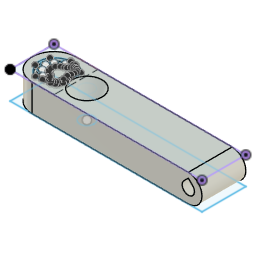
paw v9 (Autodesk Fusion 360 design; units mm, degrees)
Autodesk Fusion 360 part; units mm, degrees
note: some values were not read from the file. Set by a fixed rule: which sketch regions a step uses.
sketch "Sketch1" plane through (0, 0, 0) normal (0, 0, 1) x (1, 0, 0)
  line L0 (-0.0918, 15) -> (34.9082, 15)
  line L1 (34.9082, 15) -> (34.9082, 7)
  line L2 (34.9082, 7) -> (-0.0918, 7)
  line L3 (-0.0918, 7) -> (-0.0918, 15)
  circle A0 centre (9.9082, 11) radius 1.25
  dimension "d1" = 35
  dimension "d2" = 8
  dimension "d3" = 2.5
  dimension "d4" = 25
  dimension "d5" = 4
  constraint horizontal L0
  constraint vertical L1
  constraint horizontal L2
  constraint vertical L3
  measures "d1" distance of L0.start L0.end
  measures "d2" distance of L0.start L2.end
  measures "d3" diameter of A0
  measures "d4" distance of L1 A0.centre
  measures "d5" distance of L0 A0.centre
extrude "Extrude1" add sketch "Sketch1" along normal blind 5
sketch "Sketch2" plane through (0, 0, 5) normal (0, 0, 1) x (-1, 0, 0)
  circle A0 centre (-9.9082, -11) radius 1.25
  spline S0 degree 5 poles (-6.6668, -9.044) (-6.6524, -9.0222) (-6.6233, -8.9806) (-6.5785, -8.9237) (-6.5167, -8.8567) (-6.4345, -8.7811) (-6.3432, -8.7078) (-6.2367, -8.6364) (-6.1068, -8.5717) (-5.9478, -8.5207) (-5.758, -8.4891) (-5.5438, -8.4783) (-5.3207, -8.4835) (-5.1077, -8.496) (-4.922, -8.5058) (-4.7747, -8.5033) (-4.6652, -8.4819) (-4.5768, -8.44) (-4.4867, -8.38) (-4.3721, -8.3084) (-4.22, -8.2356) (-4.0277, -8.1741) (-3.7993, -8.1372) (-3.5437, -8.1373) (-3.272, -8.1841) (-2.9948, -8.2832) (-2.7204, -8.4347) (-2.4559, -8.635) (-2.207, -8.8773) (-1.9783, -9.1532) (-1.7741, -9.4534) (-1.5979, -9.7688) (-1.4537, -10.0915) (-1.3454, -10.416) (-1.2774, -10.7396) (-1.2539, -11.0611) (-1.2785, -11.3805) (-1.3538, -11.6979) (-1.4808, -12.0127) (-1.6588, -12.323) (-1.8844, -12.6248) (-2.1518, -12.911) (-2.4522, -13.1718) (-2.775, -13.3969) (-3.1086, -13.5764) (-3.4406, -13.7026) (-3.7589, -13.7713) (-4.0521, -13.7834) (-4.3104, -13.7462) (-4.5259, -13.6756) (-4.694, -13.5945) (-4.8153, -13.5267) (-4.8979, -13.4912) (-4.9591, -13.4967) (-5.0282, -13.5353) (-5.1366, -13.588) (-5.3079, -13.6318) (-5.5459, -13.6462) (-5.8352, -13.6163) (-6.1489, -13.5318) (-6.4539, -13.3878) (-6.7168, -13.1851) (-6.91, -12.9307) (-7.0174, -12.6376) (-7.0408, -12.3259) (-6.9955, -12.0188) (-6.9053, -11.7392) (-6.7974, -11.5057) (-6.6977, -11.3289) (-6.6262, -11.2084) (-6.5904, -11.1268) (-6.5866, -11.0551) (-6.6056, -10.9663) (-6.6389, -10.85) (-6.6814, -10.7168) (-6.7294, -10.5841) (-6.7802, -10.4678) (-6.8302, -10.3695) (-6.8748, -10.2785) (-6.9101, -10.1804) (-6.9321, -10.064) (-6.9385, -9.9273) (-6.928, -9.774) (-6.9005, -9.6117) (-6.8576, -9.4494) (-6.8023, -9.2957) (-6.7508, -9.1852) (-6.7096, -9.1111) (-6.6812, -9.0657) (-6.6668, -9.044) knots 0 0 0 0 0 0 0.01176471 0.02352941 0.03529412 0.04705882 0.05882353 0.07058824 0.08235294 0.09411765 0.10588235 0.11764706 0.12941176 0.14117647 0.15294118 0.16470588 0.17647059 0.18823529 0.2 0.21176471 0.22352941 0.23529412 0.24705882 0.25882353 0.27058824 0.28235294 0.29411765 0.30588235 0.31764706 0.32941176 0.34117647 0.35294118 0.36470588 0.37647059 0.38823529 0.4 0.41176471 0.42352941 0.43529412 0.44705882 0.45882353 0.47058824 0.48235294 0.49411765 0.50588235 0.51764706 0.52941176 0.54117647 0.55294118 0.56470588 0.57647059 0.58823529 0.6 0.61176471 0.62352941 0.63529412 0.64705882 0.65882353 0.67058824 0.68235294 0.69411765 0.70588235 0.71764706 0.72941176 0.74117647 0.75294118 0.76470588 0.77647059 0.78823529 0.8 0.81176471 0.82352941 0.83529412 0.84705882 0.85882353 0.87058824 0.88235294 0.89411765 0.90588235 0.91764706 0.92941176 0.94117647 0.95294118 0.96470588 0.97647059 0.98823529 1 1 1 1 1 1
  spline S1 degree 5 poles (-6.4128, -9.7721) (-6.4117, -9.7598) (-6.4091, -9.7361) (-6.4039, -9.7032) (-6.3944, -9.6634) (-6.3776, -9.6175) (-6.3557, -9.5726) (-6.3293, -9.5271) (-6.3006, -9.4811) (-6.272, -9.4357) (-6.245, -9.392) (-6.2194, -9.35) (-6.1921, -9.3086) (-6.1593, -9.2659) (-6.1173, -9.2203) (-6.065, -9.1713) (-6.004, -9.1201) (-5.938, -9.0687) (-5.871, -9.0197) (-5.8065, -8.9752) (-5.7462, -8.9368) (-5.6891, -8.9045) (-5.6327, -8.8778) (-5.5741, -8.856) (-5.5111, -8.8384) (-5.4437, -8.8254) (-5.3735, -8.818) (-5.3031, -8.8177) (-5.2352, -8.8263) (-5.1714, -8.845) (-5.1119, -8.8749) (-5.0556, -8.9161) (-5.0011, -8.9684) (-4.9474, -9.0305) (-4.8945, -9.1002) (-4.8437, -9.1745) (-4.7971, -9.25) (-4.7565, -9.3234) (-4.7229, -9.3922) (-4.6964, -9.4545) (-4.6745, -9.5104) (-4.6537, -9.5608) (-4.6304, -9.6073) (-4.6015, -9.6515) (-4.5655, -9.6948) (-4.5229, -9.7377) (-4.4747, -9.7804) (-4.4229, -9.8224) (-4.3695, -9.8624) (-4.3159, -9.8988) (-4.2635, -9.9302) (-4.2128, -9.9556) (-4.1634, -9.9751) (-4.1138, -9.9906) (-4.0624, -10.0044) (-4.0077, -10.0193) (-3.9495, -10.0381) (-3.8888, -10.0625) (-3.8275, -10.0939) (-3.7682, -10.1329) (-3.7131, -10.1798) (-3.6636, -10.234) (-3.6207, -10.2948) (-3.5844, -10.3613) (-3.5545, -10.4323) (-3.5305, -10.5074) (-3.5118, -10.5862) (-3.4976, -10.669) (-3.4875, -10.756) (-3.4812, -10.8475) (-3.4786, -10.9434) (-3.4805, -11.0434) (-3.4878, -11.1461) (-3.5019, -11.2502) (-3.5242, -11.3539) (-3.5559, -11.4553) (-3.5981, -11.5528) (-3.6509, -11.6448) (-3.7139, -11.7304) (-3.786, -11.809) (-3.8656, -11.8802) (-3.951, -11.944) (-4.04, -12.0007) (-4.1308, -12.0507) (-4.2216, -12.0946) (-4.3109, -12.1332) (-4.3977, -12.1673) (-4.4807, -12.1982) (-4.5594, -12.2275) (-4.6332, -12.2573) (-4.7017, -12.2898) (-4.7649, -12.3277) (-4.8227, -12.3733) (-4.8755, -12.4279) (-4.9238, -12.4918) (-4.9684, -12.5636) (-5.0103, -12.6406) (-5.0506, -12.7195) (-5.0905, -12.7966) (-5.1312, -12.8691) (-5.1741, -12.9347) (-5.2204, -12.9928) (-5.2709, -13.0432) (-5.326, -13.0864) (-5.3853, -13.1229) (-5.4475, -13.1531) (-5.5107, -13.177) (-5.5728, -13.1946) (-5.6323, -13.2053) (-5.6892, -13.2087) (-5.7449, -13.204) (-5.8018, -13.1906) (-5.8621, -13.1682) (-5.9271, -13.1368) (-5.9962, -13.0972) (-6.0672, -13.0507) (-6.1376, -12.9987) (-6.204, -12.9426) (-6.2637, -12.8837) (-6.3147, -12.8226) (-6.3562, -12.7594) (-6.3879, -12.6939) (-6.4103, -12.6259) (-6.4242, -12.5551) (-6.4307, -12.4813) (-6.4309, -12.4046) (-6.4261, -12.3254) (-6.4172, -12.244) (-6.4046, -12.1609) (-6.3882, -12.0767) (-6.3677, -11.992) (-6.3425, -11.9071) (-6.3125, -11.8224) (-6.2782, -11.7378) (-6.2411, -11.6527) (-6.204, -11.566) (-6.1704, -11.4765) (-6.1438, -11.3828) (-6.1275, -11.2837) (-6.1237, -11.1783) (-6.1334, -11.0665) (-6.1554, -10.9488) (-6.1874, -10.8263) (-6.2261, -10.7007) (-6.2675, -10.5739) (-6.3081, -10.4483) (-6.3443, -10.3261) (-6.3737, -10.2095) (-6.3953, -10.1008) (-6.4091, -10.0015) (-6.4161, -9.9131) (-6.417, -9.8514) (-6.4156, -9.81) (-6.4139, -9.7845) (-6.4128, -9.7721) knots 0 0 0 0 0 0 0.00666667 0.01333333 0.02 0.02666667 0.03333333 0.04 0.04666667 0.05333333 0.06 0.06666667 0.07333333 0.08 0.08666667 0.09333333 0.1 0.10666667 0.11333333 0.12 0.12666667 0.13333333 0.14 0.14666667 0.15333333 0.16 0.16666667 0.17333333 0.18 0.18666667 0.19333333 0.2 0.20666667 0.21333333 0.22 0.22666667 0.23333333 0.24 0.24666667 0.25333333 0.26 0.26666667 0.27333333 0.28 0.28666667 0.29333333 0.3 0.30666667 0.31333333 0.32 0.32666667 0.33333333 0.34 0.34666667 0.35333333 0.36 0.36666667 0.37333333 0.38 0.38666667 0.39333333 0.4 0.40666667 0.41333333 0.42 0.42666667 0.43333333 0.44 0.44666667 0.45333333 0.46 0.46666667 0.47333333 0.48 0.48666667 0.49333333 0.5 0.50666667 0.51333333 0.52 0.52666667 0.53333333 0.54 0.54666667 0.55333333 0.56 0.56666667 0.57333333 0.58 0.58666667 0.59333333 0.6 0.60666667 0.61333333 0.62 0.62666667 0.63333333 0.64 0.64666667 0.65333333 0.66 0.66666667 0.67333333 0.68 0.68666667 0.69333333 0.7 0.70666667 0.71333333 0.72 0.72666667 0.73333333 0.74 0.74666667 0.75333333 0.76 0.76666667 0.77333333 0.78 0.78666667 0.79333333 0.8 0.80666667 0.81333333 0.82 0.82666667 0.83333333 0.84 0.84666667 0.85333333 0.86 0.86666667 0.87333333 0.88 0.88666667 0.89333333 0.9 0.90666667 0.91333333 0.92 0.92666667 0.93333333 0.94 0.94666667 0.95333333 0.96 0.96666667 0.97333333 0.98 0.98666667 0.99333333 1 1 1 1 1 1
  ellipse E0 centre (-3.9, -9) end of major axis (-3.2, -8.7) minor radius 0.5187
  line L0 (-4.6, -9.3) -> (-3.2, -8.7) construction
  line L1 (-3.6957, -9.4768) -> (-4.1043, -8.5232) construction
  ellipse E1 centre (-2.9, -9.9) end of major axis (-3.7, -10) minor radius 0.4976
  line L2 (-2.1, -9.8) -> (-3.7, -10) construction
  line L3 (-2.9617, -9.4062) -> (-2.8383, -10.3938) construction
  ellipse E2 centre (-2.4, -11) end of major axis (-1.6, -11) minor radius 0.5
  line L4 (-3.2, -11) -> (-1.6, -11) construction
  line L5 (-2.4, -11.5) -> (-2.4, -10.5) construction
  ellipse E3 centre (-2.8652, -12.0724) end of major axis (-2.05, -12.25) minor radius 0.4956
  line L6 (-3.6805, -11.8948) -> (-2.05, -12.25) construction
  line L7 (-2.9707, -12.5567) -> (-2.7597, -11.5881) construction
  ellipse E4 centre (-4.0852, -12.9494) end of major axis (-3.3781, -13.1035) minor radius 0.4819
  line L8 (-4.7923, -12.7954) -> (-3.3781, -13.1035) construction
  line L9 (-4.1877, -13.4203) -> (-3.9826, -12.4786) construction
  line L10 (0.0918, -7) -> (-34.9082, -7)
  line L11 (-34.9082, -7) -> (-34.9082, -15)
  line L12 (-34.9082, -15) -> (0.0918, -15)
  line L13 (0.0918, -15) -> (0.0918, -7)
  line L14 (0.0918, -7) -> (-7.9082, -7) construction
  line L15 (-7.9082, -7) -> (-7.9082, -15) construction
  line L16 (-7.9082, -15) -> (0.0918, -15) construction
  line L17 (0.0918, -15) -> (0.0918, -7) construction
  point P0 (-6.3817, -8.7403)
  point P1 (-5.8, -8.5)
  point P2 (-4.8, -8.5)
  point P3 (-4.4453, -8.3552)
  point P4 (-3.3609, -8.1757)
  point P5 (-1.5203, -9.9528)
  point P6 (-1.7478, -12.4324)
  point P7 (-4.2011, -13.7562)
  point P8 (-4.9, -13.5)
  point P9 (-5.2, -13.6)
  point P10 (-6.9, -12.9)
  point P11 (-6.6668, -11.2761)
  point P12 (-6.6, -11)
  point P13 (-6.7467, -10.5475)
  point P14 (-6.9, -10.2)
  point P15 (-6.9056, -9.6556)
  point P16 (-6.3571, -9.5771)
  point P17 (-6.25, -9.4)
  point P18 (-6.1249, -9.2298)
  point P19 (-5.8166, -8.9828)
  point P20 (-5.55, -8.85)
  point P21 (-5.2371, -8.8286)
  point P22 (-4.9641, -9.0125)
  point P23 (-4.7226, -9.3951)
  point P24 (-4.6223, -9.618)
  point P25 (-4.45, -9.8)
  point P26 (-4.2211, -9.9504)
  point P27 (-4.0168, -10.0173)
  point P28 (-3.75, -10.15)
  point P29 (-3.55, -10.45)
  point P30 (-3.48, -10.9144)
  point P31 (-3.6, -11.55)
  point P32 (-4.0725, -12.0177)
  point P33 (-4.5722, -12.2331)
  point P34 (-4.8805, -12.4374)
  point P35 (-5.1126, -12.8349)
  point P36 (-5.35, -13.1)
  point P37 (-5.6253, -13.2026)
  point P38 (-5.8686, -13.1636)
  point P39 (-6.2233, -12.9222)
  point P40 (-6.4128, -12.6064)
  point P41 (-6.4128, -12.2183)
  point P42 (-6.2828, -11.7502)
  point P43 (-6.1267, -11.1949)
  point P44 (-6.35, -10.3)
  dimension "d38" = 8
  constraint coincident E0 L0.start
  constraint coincident E0 L0.end
  constraint coincident E0 L1.start
  constraint coincident E0 L1.end
  constraint coincident E1 L2.start
  constraint coincident E1 L2.end
  constraint coincident E1 L3.start
  constraint coincident E1 L3.end
  constraint coincident E2 L4.start
  constraint coincident E2 L4.end
  constraint coincident E2 L5.start
  constraint coincident E2 L5.end
  constraint horizontal L4
  constraint coincident E3 L6.start
  constraint coincident E3 L6.end
  constraint coincident E3 L7.start
  constraint coincident E3 L7.end
  constraint coincident E4 L8.start
  constraint coincident E4 L8.end
  constraint coincident E4 L9.start
  constraint coincident E4 L9.end
  constraint perpendicular L7 L8
  constraint horizontal L14
  constraint vertical L15
  constraint horizontal L16
  constraint vertical L17
  constraint coincident L10.start L13.end
  measures "d38" distance of L10.start L14.end
sketch "Sketch6" plane through (0, 7, 0) normal (0, -1, 0) x (1, 0, 0)
  line L0 (-0.0918, 0) -> (34.9082, 0)
  line L1 (34.9082, 0) -> (34.9082, 5)
  line L2 (34.9082, 5) -> (-0.0918, 5)
  line L3 (-0.0918, 5) -> (-0.0918, 0)
  line L4 (34.9082, 5) -> (29.9082, 5) construction
  line L5 (29.9082, 5) -> (29.9082, 0) construction
  line L6 (29.9082, 0) -> (34.9082, 0) construction
  line L7 (34.9082, 0) -> (34.9082, 5) construction
  line L8 (33.5332, 2.5) -> (31.2832, 2.5) construction
  line L9 (31.521, 3.1917) -> (31.7298, 3.1917) construction
  line L10 (31.7166, 3.3873) -> (32.4145, 4.0789)
  line L11 (32.4145, 4.0789) -> (33.0999, 3.3873)
  arc A0 (31.7166, 3.3873) -> (33.0999, 3.3873) centre (32.4082, 2.5) ccw
  dimension "d47" = 5
  dimension "d48" = 5
  dimension "d49" = 2.25
  constraint horizontal L4
  constraint vertical L5
  constraint horizontal L6
  constraint vertical L7
  constraint coincident L1.end L2.start
  constraint coincident L8.start A0
  constraint coincident L8.end A0
  constraint perpendicular L7 L8
  constraint horizontal L9
  constraint coincident L9.start A0
  constraint perpendicular L10 L11
  measures "d47" distance of L1.end L4.end
  measures "d48" distance of L1.end L0.end
  measures "d49" diameter of A0
extrude "Extrude9" cut sketch "Sketch6" against normal blind 8 contours L10 L11 A0
fillet "Fillet8" radius 2.5 2 edges at (34.9082, 11, 5) (34.9082, 11, 0)
fillet "Fillet9" radius 4 2 edges at (-0.0918, 15, 2.5) (-0.0918, 7, 2.5)
extrude "Extrude10" cut sketch "Sketch2" against normal blind 0.5 contours S0
chamfer "Chamfer1" distance 1.5 angle 70 1 edges at (8.7428, 11.452, 5) measured on face at (25.3252, 11, 5)
